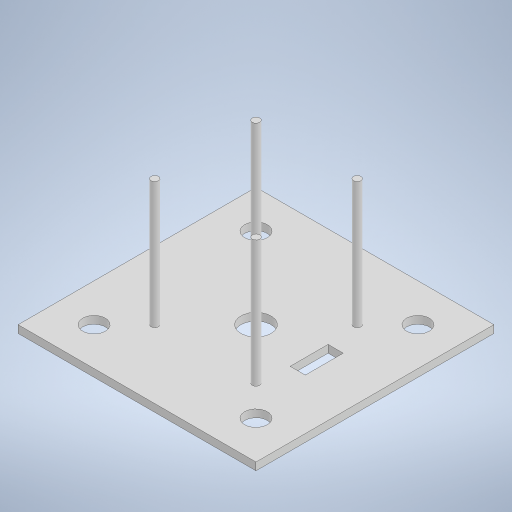
# Autodesk Inventor part: Button Plate
Saved by Autodesk Inventor 2024.1 (Build 281209000, 209)
## iProperties
Created: 2023-12-23
Part Number: Button Plate
Material: Generic
Document SubType Name: Modeling
Designer: ryanm
Density: 1 g/cm^3
Appearance: Default
Author: ryanm
Autodesk Inventor part; units mm, degrees
ref_plane "YZ Plane" through (0, 0, 0) normal (1, 0, 0) x (0, 1, 0)
ref_plane "XZ Plane" through (0, 0, 0) normal (0, 1, 0) x (-1, 0, 0)
ref_plane "XY Plane" through (0, 0, 0) normal (0, 0, 1) x (1, 0, 0)
sketch "Sketch1" plane through (0, 0, 0) normal (0, 1, 0) x (-1, 0, 0)
  line L0 (47, -47) -> (-47, -47)
  line L1 (-47, -47) -> (-47, 47)
  line L2 (-47, 47) -> (47, 47)
  line L3 (47, 47) -> (47, -47)
  point P0 (0, 0)
  point P1 (0, -47)
  point P2 (47, 0)
  dimension "d0" = 94
  dimension "d1" = 94
  constraints: 8 end point, 2 midpoint, 2 parallel, 1 horizontal, 1 horizontal alignment, 1 perpendicular, 1 vertical alignment
  measures "d0" distance of L0.start L0.end
  measures "d1" distance of L2.end L0.start
extrude "Extrusion1" add sketch "Sketch1" along normal blind 3
sketch "Sketch2" plane through (0, 3, 0) normal (0, 1, 0) x (1, 0, 0)
  circle A0 centre (0, 0) radius 6
  dimension "d4" = 12
  constraints: 1 centre point, 1 coincident
  measures "d4" diameter of A0
extrude "Extrusion2" cut sketch "Sketch2" against normal through all
sketch "Sketch3" plane through (0, 3, 0) normal (0, 1, 0) x (1, 0, 0)
  circle A0 centre (-32, 32) radius 4.5
  circle A1 centre (32, 32) radius 4.5
  circle A2 centre (32, -32) radius 4.5
  circle A3 centre (-32, -32) radius 4.5
  line L0 (47, 47) -> (-47, 47) projected
  line L1 (-47, 47) -> (-47, -47) projected
  line L2 (47, -47) -> (47, 47) projected
  line L3 (-47, -47) -> (47, -47) projected
  point P0 (0, 0)
  dimension "d7" = 9
  dimension "d8" = 9
  dimension "d9" = 9
  dimension "d10" = 9
  dimension "d11" = 15
  dimension "d12" = 15
  dimension "d13" = 15
  dimension "d14" = 15
  constraints: 4 centre point, 2 horizontal alignment, 2 vertical alignment
  measures "d7" diameter of A0
  measures "d8" diameter of A1
  measures "d9" diameter of A2
  measures "d10" diameter of A3
  measures "d11" distance from line of L0 A0.centre
  measures "d12" distance from line of L1 A0.centre
  measures "d13" distance from line of L2 A2.centre
  measures "d14" distance from line of L3 A2.centre
extrude "Extrusion3" cut sketch "Sketch3" against normal through all contours A0 | A1 | A2 | A3
sketch "Sketch4" plane through (0, 3, 0) normal (0, 1, 0) x (1, 0, 0)
  circle A0 centre (-20, 20) radius 1.5
  circle A1 centre (20, 20) radius 1.5
  circle A2 centre (20, -20) radius 1.5
  circle A3 centre (-20, -20) radius 1.5
  point P0 (0, 0)
  dimension "d17" = 3
  dimension "d18" = 3
  dimension "d19" = 3
  dimension "d20" = 3
  dimension "d21" = 20
  dimension "d22" = 20
  dimension "d23" = 20
  dimension "d24" = 20
  constraints: 4 centre point, 2 horizontal alignment, 2 vertical alignment
  measures "d17" diameter of A0
  measures "d18" diameter of A1
  measures "d19" diameter of A2
  measures "d20" diameter of A3
  measures "d21" horizontal distance of A1.centre point (0, 0)
  measures "d22" horizontal distance of A0.centre point (0, 0)
  measures "d23" horizontal distance of A0.centre point (0, 0)
  measures "d24" horizontal distance of A3.centre point (0, 0)
extrude "Extrusion4" add sketch "Sketch4" along normal blind 50
sketch "Sketch5" plane through (0, 3, 0) normal (0, 1, 0) x (1, 0, 0)
  line L0 (21, 7.5) -> (27, 7.5)
  line L1 (27, 7.5) -> (27, -7.5)
  line L2 (27, -7.5) -> (21, -7.5)
  line L3 (21, -7.5) -> (21, 7.5)
  line L4 (47, -47) -> (47, 47) projected
  point P0 (0, 0)
  point P1 (21, 0)
  dimension "d27" = 15
  dimension "d28" = 6
  dimension "d29" = 20
  constraints: 8 end point, 2 parallel, 1 horizontal, 1 horizontal alignment, 1 midpoint, 1 perpendicular
  measures "d27" distance of L0.end L1.end
  measures "d28" distance of L0.start L0.end
  measures "d29" distance between parallel lines of L4 L1
extrude "Extrusion5" cut sketch "Sketch5" against normal through all
equation "\"d8\" = d7"
equation "\"d9\" = d7"
equation "\"d10\" = d7"
equation "\"d13\" = d12"
equation "\"d14\" = d11"
equation "\"d22\" = d21"
equation "\"d23\" = d22"
equation "\"d24\" = d22"
body "Solid1"
